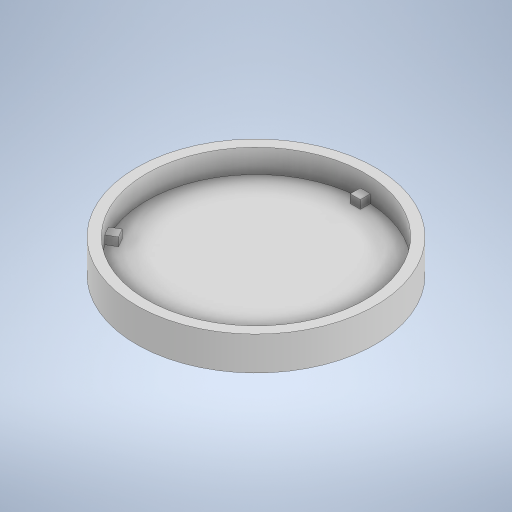
# Autodesk Inventor part: Orchid Coaster V1
Saved by Autodesk Inventor 2024 (Build 280153000, 153)
## iProperties
Created: 2024-02-28
Part Number: Orchid Coaster V1
Material: Generic
Document SubType Name: Modeling
Designer: haque
Density: 1 g/cm^3
Appearance: Default
Author: haque
Autodesk Inventor part; units mm, degrees
ref_plane "YZ Plane" through (0, 0, 0) normal (1, 0, 0) x (0, 1, 0)
ref_plane "XZ Plane" through (0, 0, 0) normal (0, 1, 0) x (-1, 0, 0)
ref_plane "XY Plane" through (0, 0, 0) normal (0, 0, 1) x (1, 0, 0)
sketch "Sketch1" plane through (0, 0, 0) normal (0, 1, 0) x (-1, 0, 0)
  circle A0 centre (0, 0) radius 32.5
  circle A1 centre (0, 0) radius 35.5
  dimension "d0" = 65
  dimension "d1" = 71
  constraints: 2 centre point, 2 coincident
  measures "d0" diameter of A0
  measures "d1" diameter of A1
extrude "Extrusion1" add sketch "Sketch1" along normal blind 10
extrude "Extrusion2" add sketch "Sketch1" along normal blind 3 contours A0
sketch "Sketch2" plane through (0, 3, 0) normal (0, 1, 0) x (1, 0, 0)
  circle A0 centre (0, 0) radius 32.5 projected
  line L0 (0, 32.5) -> (0, 29.5)
  line L1 (-1.5, 29.5) -> (-1.5, 32.5)
  line L2 (-1.5, 32.5) -> (1.5, 32.5)
  line L3 (1.5, 32.5) -> (1.5, 29.5)
  line L4 (1.5, 29.5) -> (-1.5, 29.5)
  line L5 (-1.5, 29.5) -> (1.5, 32.5) construction
  line L6 (-1.5, 32.5) -> (1.5, 29.5) construction
  point P0 (0, 31)
  point P1 (1.5, 32.4654)
  point P2 (-1.5, 32.4654)
  dimension "d7" = 3
  dimension "d8" = 3
  constraints: 14 end point, 3 midpoint, 3 parallel, 1 perpendicular, 1 vertical, 2 other
  measures "d7" distance of L0.start L0.end
  measures "d8" distance of L1.end L2.end
extrude "Extrusion3" add sketch "Sketch2" along normal blind 2.5 contours L3 L4 L0 A0 | A0 L0 L4 L1
pattern_circular "Circular Pattern1" count 3 over 360 about axis through (0, -10, 0) along (0, 1, 0) of "Extrusion3"
body "Solid1"
